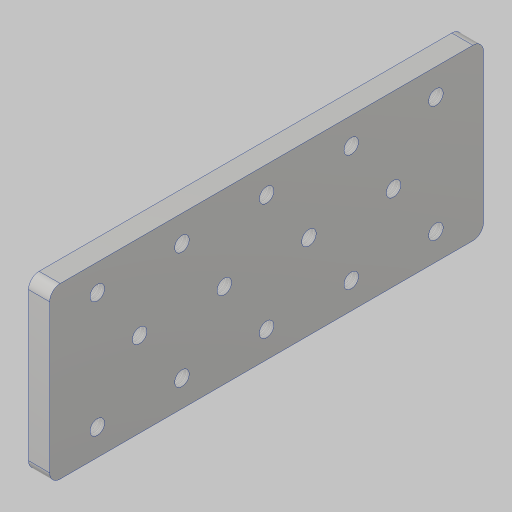
# Autodesk Inventor part: CL4-021
Saved by Autodesk Inventor 2023.5 (Build 275446000, 446)
## iProperties
Created: 2025-02-09
Part Number: CL4-021
Material: Aluminum 6061
Document SubType Name: Modeling
Designer: slick
Density: 2.7 g/cm^3
Appearance: Aluminum - Flat
Author: slick
Autodesk Inventor part; units mm, degrees
note: some values were not read from the file. Chosen so that the rebuilt part matches the saved one: second side of "Extrusion1".
ref_plane "YZ Plane" through (0, 0, 0) normal (1, 0, 0) x (0, 1, 0)
ref_plane "XZ Plane" through (0, 0, 0) normal (0, 1, 0) x (-1, 0, 0)
ref_plane "XY Plane" through (0, 0, 0) normal (0, 0, 1) x (1, 0, 0)
sketch "Sketch1" plane through (0, 0, 0) normal (1, 0, 0) x (0, 1, 0)
  line L0 (-25.4, -65.0875) -> (25.4, -65.0875)
  line L1 (25.4, -65.0875) -> (25.4, 65.0875)
  line L2 (25.4, 65.0875) -> (-25.4, 65.0875)
  line L3 (-25.4, 65.0875) -> (-25.4, -65.0875)
  line L4 (-25.4, -65.0875) -> (25.4, 65.0875) construction
  line L5 (25.4, -65.0875) -> (-25.4, 65.0875) construction
  point P0 (0, 0)
  dimension "d0" = 130.175
  dimension "d1" = 50.8
  constraints: 12 end point, 2 midpoint, 2 parallel, 1 horizontal, 1 perpendicular
  measures "d0" distance of L0.end L1.end
  measures "d1" distance of L1.end L2.end
extrude "Extrusion1" add sketch "Sketch1" along normal blind 6.35
sketch "Sketch2" plane through (6.35, 0, 0) normal (1, 0, 0) x (0, 0, -1)
  line L0 (-50.8, 17.4625) -> (-50.8, -17.4625) construction
  line L1 (-65.0875, 25.4) -> (-65.0875, -25.4) construction
  line L2 (65.0875, 25.4) -> (65.0875, -25.4) construction
  line L3 (65.0875, -25.4) -> (-65.0875, -25.4) construction
  line L4 (-65.0875, 25.4) -> (65.0875, 25.4) construction
  line L5 (-65.0875, -25.4) -> (-65.0875, 25.4) projected
  point P0 (0, 0)
  point P1 (-38.1, 0)
  point P2 (-50.8, 0)
  point P3 (-65.0875, 0)
  point P4 (-25.4, 17.4625)
  point P5 (-12.7, 0)
  point P6 (-25.4, -17.4625)
  point P7 (0, 17.4625)
  point P8 (12.7, 0)
  point P9 (0, -17.4625)
  point P10 (25.4, 17.4625)
  point P11 (38.1, 0)
  point P12 (25.4, -17.4625)
  point P13 (50.8, 17.4625)
  point P14 (63.5, 0)
  point P15 (50.8, -17.4625)
  dimension "d6" = 34.925
  dimension "d7" = 14.2875
  dimension "d8" = 12.7
  dimension "d11" = 25.4
  constraints: 2 end point, 2 horizontal alignment, 2 midpoint, 1 horizontal, 1 vertical, 1 vertical alignment, 12 other
  measures "d6" distance of L0.start L0.end
  measures "d7" distance from line of L1 L0.start
  measures "d8" horizontal distance of point (-38.1, 0) L0.start
  measures "d11" distance of L0.start point (-25.4, 17.462)
hole "Hole1" at (6.35, -17.4625, 50.8) at (6.35, 17.4625, 50.8) at (6.35, 0, 38.1) at (6.35, 17.4625, 25.4) at (6.35, 0, 12.7) at (6.35, -17.4625, 25.4) at (6.35, 17.4625, 0) at (6.35, 0, -12.7) at (6.35, -17.4625, 0) at (6.35, 17.4625, -25.4) at (6.35, -17.4625, -25.4) at (6.35, 0, -38.1) at (6.35, 17.4625, -50.8) at (6.35, -17.4625, -50.8) direction (-1, 0, 0) diameter 4.3434 end through all thread size "12-24 UNC" class "2B" standard "ANSI Unified Screw Threads"
fillet "Fillet1" radius 3.175 4 edges at (3.175, 25.4, 65.0875) (3.175, 25.4, -65.0875) (3.175, -25.4, -65.0875) (3.175, -25.4, 65.0875)
body "Solid1"
